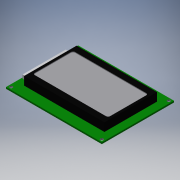
# Autodesk Inventor part: Grøn PCB
Saved by Autodesk Inventor 2016 (Build 200138000, 138)
## iProperties
Created: 2015-06-10
Part Number: Grøn PCB
Material: Generic
Document SubType Name: Modeling
Designer: Mathias L. Kjeldgaard
Density: 1 g/cm^3
Appearance: Default
Author: Mathias L. Kjeldgaard
Autodesk Inventor part; units mm, degrees
ref_plane "YZ Plane" through (0, 0, 0) normal (1, 0, 0) x (0, 1, 0)
ref_plane "XZ Plane" through (0, 0, 0) normal (0, 1, 0) x (-1, 0, 0)
ref_plane "Work Plane1" through (0, 0, 2.54) normal (0, 0, 1) x (1, 0, 0)
sketch "Sketch2" plane through (0, 0, 2.54) normal (0, 0, 1) x (1, 0, 0)
  line L0 (6.5, -32.5) -> (6.5, -38.5) projected
  line L1 (6.5, -38.5) -> (0.5, -38.5) projected
  line L2 (0.5, -38.5) -> (0.5, -32.5) projected
  line L3 (0.5, -32.5) -> (6.5, -32.5) projected
  circle A0 centre (19.75, -34.75) radius 5.75 projected
  line L4 (43.5, -29) -> (43.5, -41.5) projected
  line L5 (43.5, -41.5) -> (30, -41.5) projected
  line L6 (30, -41.5) -> (30, -29) projected
  line L7 (30, -29) -> (43.5, -29) projected
  circle A1 centre (44, 41) radius 1.5 projected
  circle A2 centre (-44, 41) radius 1.5 projected
  line L8 (46.5, 43.5) -> (-46.5, 43.5) projected
  line L9 (-46.5, 43.5) -> (-46.5, -43.5) projected
  line L10 (-46.5, -43.5) -> (46.5, -43.5) projected
  line L11 (46.5, -43.5) -> (46.5, 43.5) projected
  line L12 (-46.5, 43.5) -> (46.5, 43.5)
  line L13 (46.5, 43.5) -> (46.5, -26.5)
  line L14 (46.5, -26.5) -> (-46.5, -26.5)
  line L15 (-46.5, -26.5) -> (-46.5, 43.5)
  circle A3 centre (-44, 41) radius 1.5
  circle A4 centre (44, 41) radius 1.5
  circle A5 centre (44, -24) radius 1.5
  circle A6 centre (-44, -24) radius 1.5
  line L16 (-45.5, -20.479) -> (-45.5, -25.5) construction
  line L17 (-45.5, -25.5) -> (-36.292, -25.5) construction
  line L18 (45.5, -16.7483) -> (45.5, -25.5) construction
  line L19 (45.5, -25.5) -> (38.0013, -25.5) construction
  circle A7 centre (-44, -24) radius 1.5 projected
  circle A8 centre (44, -24) radius 1.5 projected
  point P0 (0, 0)
  dimension "d0" = 70
  dimension "d1" = 3
  dimension "d2" = 3
  dimension "d3" = 1
  dimension "d4" = 1
  dimension "d5" = 1
  dimension "d6" = 1
  dimension "d21" = 65
  dimension "d22" = 65
  constraints: 16 end point, 4 centre point, 4 perpendicular, 4 tangent, 3 parallel, 2 coincident, 2 concentric, 1 horizontal, 1 point on line
  measures "d0" distance between parallel lines of L12 L14
  measures "d1" diameter of A5
  measures "d2" diameter of A6
  measures "d3" distance between parallel lines of L14 L17
  measures "d4" distance between parallel lines of L15 L16
  measures "d5" distance between parallel lines of L13 L18
  measures "d6" distance between parallel lines of L14 L19
  measures "d21" distance of A2.centre A6.centre
  measures "d22" distance of A5.centre A1.centre
extrude "Tykkelsen Grøn PCB" add sketch "Sketch2" along normal blind 1.5 contours L11 L14 L9 L8
sketch "Sketch3" plane through (0, 0, 4.04) normal (0, 0, 1) x (1, 0, 0)
  line L0 (-46.5, 43.5) -> (-46.5, -26.5) projected
  line L1 (46.5, -26.5) -> (46.5, 43.5) projected
  line L2 (46.5, 43.5) -> (-46.5, 43.5) projected
  line L3 (-39, 34.5) -> (39, 34.5)
  line L4 (39, 34.5) -> (39, -16.5)
  line L5 (39, -16.5) -> (-39, -16.5)
  line L6 (-39, -16.5) -> (-39, 34.5)
  point P0 (0, 0)
  dimension "d9" = 51
  dimension "d10" = 78
  dimension "d11" = 7.5
  dimension "d12" = 7.5
  dimension "d13" = 9
  constraints: 8 end point, 2 parallel, 1 horizontal, 1 perpendicular
  measures "d9" distance of L3.end L4.end
  measures "d10" distance of L4.end L5.end
  measures "d11" distance between parallel lines of L1 L4
  measures "d12" distance between parallel lines of L0 L6
  measures "d13" distance between parallel lines of L2 L3
extrude "Skærm" add sketch "Sketch3" along normal blind 8
sketch "Sketch5" plane through (0, 0, 12.04) normal (0, 0, 1) x (1, 0, 0)
  line L0 (39, 34.5) -> (-39, 34.5) projected
  line L1 (-39, 34.5) -> (-39, -16.5) projected
  line L2 (-39, -16.5) -> (39, -16.5) projected
  line L3 (39, -16.5) -> (39, 34.5) projected
  line L4 (-34.5, 28.5) -> (34.5, 28.5)
  line L5 (36.5, 26.5) -> (36.5, -8.5)
  line L6 (34.5, -10.5) -> (-34.5, -10.5)
  line L7 (-36.5, -8.5) -> (-36.5, 26.5)
  arc A0 (-34.5, 28.5) -> (-36.5, 26.5) centre (-34.5, 26.5) ccw
  arc A1 (36.5, 26.5) -> (34.5, 28.5) centre (34.5, 26.5) ccw
  arc A2 (34.5, -10.5) -> (36.5, -8.5) centre (34.5, -8.5) ccw
  arc A3 (-36.5, -8.5) -> (-34.5, -10.5) centre (-34.5, -8.5) ccw
  point P0 (0, 0)
  dimension "d23" = 2.5
  dimension "d24" = 6
  dimension "d25" = 2.5
  dimension "d26" = 6
  dimension "d27" = 2
  constraints: 8 end point, 8 point on circle, 8 tangent, 4 centre point, 3 equal radius, 2 parallel, 1 horizontal, 1 perpendicular
  measures "d23" distance between parallel lines of L3 L5
  measures "d24" distance between parallel lines of L0 L4
  measures "d25" distance between parallel lines of L1 L7
  measures "d26" distance between parallel lines of L2 L6
  measures "d27" radius of A0
extrude "Hul ned i skærm" cut sketch "Sketch5" against normal blind 0.7 contours L4 A1 L5 A2 L6 A3 L7 A0
sketch "Sketch4" plane through (0, 0, 4.04) normal (0, 0, 1) x (1, 0, 0)
  line L0 (-39, -16.5) -> (-39, 34.5) projected
  line L1 (-39, 34.5) -> (39, 34.5) projected
  line L2 (-45.5, 30.5) -> (-39, 30.5)
  line L3 (-39, 30.5) -> (-39, -11.5)
  line L4 (-39, -11.5) -> (-45.5, -11.5)
  line L5 (-45.5, -11.5) -> (-45.5, 30.5)
  point P0 (0, 0)
  dimension "d16" = 42
  dimension "d17" = 6.5
  dimension "d18" = 4
  constraints: 8 end point, 2 parallel, 1 horizontal, 1 perpendicular, 1 point on line
  measures "d16" distance between parallel lines of L2 L4
  measures "d17" distance between parallel lines of L3 L5
  measures "d18" distance between parallel lines of L1 L2
extrude "Hvid ting" add sketch "Sketch4" along normal blind 3.5
equation "\"d11\" = d12"
body "Solid1"
